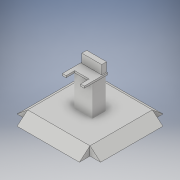
# Autodesk Inventor part: terminal stand removed rails 2nd map
Saved by Autodesk Inventor 2017 (Build 210142000, 142)
## iProperties
Created: 2018-03-07
Part Number: terminal stand removed rails 2nd map
Material: Generic
Document SubType Name: Modeling
Designer: Braxton
Density: 1 g/cm^3
Appearance: Default
Author: Braxton
Autodesk Inventor part; units mm, degrees
ref_plane "YZ Plane" through (0, 0, 0) normal (1, 0, 0) x (0, 1, 0)
ref_plane "bottom workplane" through (0, 0, 0) normal (0, 1, 0) x (-1, 0, 0)
ref_plane "XY Plane" through (0, 0, 0) normal (0, 0, 1) x (1, 0, 0)
sketch "bace of terminal" plane through (0, 0, 0) normal (0, 1, 0) x (-1, 0, 0)
  ellipse E0 centre (0, 0) end of major axis (25.4, 0) minor radius 19.05 construction
  line L0 (25.4, -19.05) -> (-25.4, -19.05)
  line L1 (-25.4, -19.05) -> (-25.4, 19.05)
  line L2 (-25.4, 19.05) -> (25.4, 19.05)
  line L3 (25.4, 19.05) -> (25.4, -19.05)
  point P0 (0, -19.05)
  dimension "d0" = 25.4
  dimension "d1" = 19.05
  constraints: 8 end point, 3 horizontal, 2 parallel, 2 vertical, 1 coincident, 1 perpendicular, 1 vertical alignment, 2 other
extrude "Extrusion16" add sketch "bace of terminal" along normal blind 92.6924
sketch "Sketch23" plane through (0, 92.6924, 0) normal (0, 1, 0) x (1, 0, 0)
  line L0 (0, 24.0896) -> (0, -74.4773) construction
  line L1 (-20.6375, -23.0226) -> (-31.2208, -23.0226) construction
  ellipse E0 centre (6.1023, 2.4529) end of major axis (37.558, 2.4529) minor radius 23.5917 (-25.2105, 0.2068) -> (-25.2085, 0.1915) ccw
  line L2 (20.6375, -23.0226) -> (31.2208, -23.0226) construction
  ellipse E1 centre (6.1023, 2.4529) end of major axis (-295.2488, 5.3941) minor radius 21.5528 (-0.0869, -19.0363) -> (0, -19.0372) ccw
  ellipse E2 centre (0, 0) end of major axis (25.3978, 0.4439) minor radius 19.0477
  line L3 (-25.9292, -47.625) -> (-25.9292, -19.05) construction
  line L4 (-25.9292, -19.05) -> (25.9292, -19.05) construction
  line L5 (3.3247, -11.6902) -> (-3.3534, -11.6902)
  line L6 (31.2208, 19.05) -> (-31.2208, 19.05)
  line L7 (-31.2208, 19.05) -> (-31.2208, -23.0226)
  line L8 (-25.4, 19.05) -> (-25.4, -19.05) projected
  line L9 (25.4, 19.05) -> (-25.4, 19.05) projected
  line L10 (25.4, -19.05) -> (25.4, 19.05) projected
  line L11 (-25.4, -19.05) -> (25.4, -19.05) projected
  line L12 (31.2208, -23.0226) -> (31.2208, 19.05)
  line L13 (-31.2208, -23.0226) -> (-31.2208, -47.625)
  line L14 (-31.2208, -47.625) -> (-20.6375, -47.625)
  line L15 (-20.6375, -47.625) -> (-20.6375, -23.0226)
  line L16 (31.2208, -23.0226) -> (31.2208, -47.625)
  line L17 (31.2208, -47.625) -> (20.6375, -47.625)
  line L18 (20.6375, -47.625) -> (20.6375, -23.0226)
  line L19 (-20.6375, -23.0226) -> (20.6375, -23.0226)
  point P0 (22.5643, 8.9693)
  dimension "d163" = 20.6375
  dimension "d165" = 10.5833
  dimension "d166" = 20.6375
  dimension "d167" = 10.5833
  dimension "d175" = 28.575
  dimension "d234" = 3.9726
  constraints: 32 end point, 9 vertical, 6 perpendicular, 5 horizontal, 4 collinear, 1 coincident, 1 midpoint, 1 point on line, 10 other
  measures "d163" distance from line of L1.start L0
  measures "d165" distance of L1.start L1.end
  measures "d166" distance from line of L2.start L0
  measures "d167" distance of L2.start L2.end
  measures "d175" distance of L3.start L3.end
  measures "d234" distance between parallel lines of L11 L1
extrude "arm rests and terminal monitor" add sketch "Sketch23" along normal blind 5.2917 separate body
ref_plane "middle of the part vertical" through (0, 0, 19.05) normal (1, 0, 0) x (0, 0, -1)
sketch "used to line up the key board and mouse" plane through (0, 97.984, 0) normal (0, 1, 0) x (1, 0, 0)
  line L0 (-25.9292, -46.3435) -> (-25.9292, -17.7685)
  line L1 (-25.9292, -17.7685) -> (25.9292, -17.7685) construction
  line L2 (25.9292, -46.1769) -> (25.9292, -17.7685)
  line L3 (-20.6375, -23.0226) -> (20.6375, -23.0226) projected
  point P0 (0, 0)
  dimension "d170" = 28.575
  dimension "d235" = 5.2541
  constraints: 6 end point, 1 horizontal, 1 perpendicular
  measures "d170" distance of L0.start L0.end
  measures "d235" distance between parallel lines of L3 L1
sketch "Sketch15" plane through (0, 0, 0) normal (0, -1, 0) x (1, 0, 0)
  line L0 (88.9, 88.9) -> (-88.9, 88.9)
  line L1 (-88.9, 88.9) -> (-88.9, -88.9)
  line L2 (-88.9, -88.9) -> (88.9, -88.9)
  line L3 (88.9, -88.9) -> (88.9, 88.9)
  line L4 (88.9, 0) -> (-88.9, 0) construction
  point P0 (0, 0)
  point P1 (0, 0)
  dimension "d236" = 177.8
  dimension "d237" = 177.8
  constraints: 10 end point, 3 midpoint, 2 parallel, 1 coincident, 1 horizontal, 1 perpendicular
  measures "d236" distance of L2.end L1.end
  measures "d237" distance of L1.end L0.end
extrude "bace" add sketch "Sketch15" along normal blind 25.4 bodies 2
sketch "Sketch31" plane through (88.9, 0, 88.9) normal (1, 0, 0) x (0, 0, -1)
  line L0 (0, 0) -> (0, -25.4) projected
  line L1 (0, 0) -> (0, -25.4)
  line L2 (0, -25.4) -> (-30.2705, -25.4)
  line L3 (-30.2705, -25.4) -> (0, 0)
  point P0 (88.9, 0)
  dimension "d238" = 40
  constraints: 6 end point, 1 perpendicular, 1 vertical
  measures "d238" angle of L2 L3
extrude "ramp to terminal" add sketch "Sketch31" against normal up to surface (177.8 mm away) bodies 2
pattern_circular "made rest of ramps to terminal" count 4 over 360 about axis through (0, -10, 0) along (0, 1, 0) of "ramp to terminal" bodies 2
ref_plane "mate to back to monitor" through (25.4, 0, -19.05) normal (0, 0, -1) x (-1, 0, 0)
sketch "Sketch25" plane through (0, 97.984, 0) normal (0, 1, 0) x (1, 0, 0)
  line L0 (0, 0) -> (0, 12.0948) construction
  line L1 (-31.2208, 19.05) -> (31.2208, 19.05) projected
  line L2 (28.3394, 5.0104) -> (-28.3394, 5.0104)
  line L3 (-28.3394, 5.0104) -> (-28.3394, 19.05)
  line L4 (-28.3394, 19.05) -> (28.3394, 19.05)
  line L5 (28.3394, 19.05) -> (28.3394, 5.0104)
  point P0 (0, 5.0104)
  dimension "d245" = 14.0396
  dimension "d246" = 56.6788
  dimension "d247" = 2.8814
  constraints: 10 end point, 2 parallel, 2 point on line, 1 horizontal, 1 perpendicular, 1 vertical
  measures "d245" distance of L4.end L2.start
  measures "d246" distance of L2.start L2.end
  measures "d247" distance from line of L1.end L5
extrude "monitor raise" add sketch "Sketch25" along normal blind 25.4 bodies 2
sketch "Sketch26" plane through (0, 0, 0) normal (0, 1, 0) x (1, 0, 0)
  line L0 (-2.9432, 29.9138) -> (2.9432, 29.9138)
  line L1 (2.9432, 29.9138) -> (2.9432, 20.32)
  line L2 (2.9432, 20.32) -> (-2.9432, 20.32)
  line L3 (-2.9432, 20.32) -> (-2.9432, 29.9138)
  line L4 (0, 19.05) -> (0, 20.32) construction
  line L5 (0, 0) -> (0, 19.05) construction
  line L6 (-25.4, 19.05) -> (25.4, 19.05) projected
  line L7 (25.4, -19.05) -> (-25.4, -19.05) projected
  line L8 (-25.4, 19.05) -> (25.4, 19.05)
  line L9 (25.4, 19.05) -> (25.4, -19.05)
  line L10 (25.4, -19.05) -> (-25.4, -19.05)
  line L11 (-25.4, -19.05) -> (-25.4, 19.05)
  line L12 (-25.4, 0) -> (0, 0)
  line L13 (0, 0) -> (0, -19.05)
  dimension "d182" = 5.8864
  dimension "d183" = 9.5938
  dimension "d185" = 1.27
  constraints: 24 end point, 4 midpoint, 4 parallel, 3 horizontal, 3 perpendicular, 2 vertical
  measures "d182" distance of L1.end L2.end
  measures "d183" distance of L0.end L1.end
  measures "d185" distance from line of L2 L4.start
ref_plane "Work Plane20" through (0, 0.4604, 0) normal (0, 1, 0) x (1, 0, 0)
sketch "Sketch27" plane through (0, 0.4604, 0) normal (0, 1, 0) x (1, 0, 0)
  line L0 (-2.4913, 29.4619) -> (2.4913, 29.4619)
  line L1 (2.4913, 29.4619) -> (2.4913, 20.7719)
  line L2 (2.4913, 20.7719) -> (-2.4913, 20.7719)
  line L3 (-2.4913, 20.7719) -> (-2.4913, 29.4619)
  line L4 (0, 0) -> (0, 19.05)
  line L5 (0, 19.05) -> (0, 20.7719) construction
  line L6 (-25.4, 19.05) -> (25.4, 19.05) projected
  point P0 (-25.4, 0)
  point P1 (-6.6832, 19.05)
  dimension "d186" = 1.7219
  dimension "d188" = 4.9826
  dimension "d189" = 8.69
  constraints: 12 end point, 2 midpoint, 2 parallel, 2 perpendicular, 1 coincident, 1 collinear, 1 horizontal, 1 point on line, 1 other
  measures "d186" distance from line of L2 L4.end
  measures "d188" distance between parallel lines of L1 L3
  measures "d189" distance between parallel lines of L2 L0
loft "outlet cap" add profiles "Sketch26", "Sketch27" bodies 2 contours L0 L1 L2 L3 / all
sketch "Sketch28" plane through (-2.4913, 0.4604, -29.4619) normal (0, 1, 0) x (1, 0, 0)
  line L0 (2.4913, -0.7892) -> (3.265, -0.7892)
  line L1 (2.4913, -3.1536) -> (3.265, -3.1536)
  arc A0 (3.265, -3.1536) -> (3.265, -0.7892) centre (2.4868, -1.9714) ccw
  line L2 (2.4913, -0.7892) -> (2.4913, -3.1536) construction
  line L3 (0, 0) -> (4.9826, 0) projected
  line L4 (2.4913, 0) -> (2.4913, 1.3195) construction
  line L5 (2.4913, -0.7892) -> (1.7177, -0.7892)
  line L6 (2.4913, -3.1536) -> (1.7177, -3.1536)
  arc A1 (1.7177, -0.7892) -> (1.7177, -3.1536) centre (2.4959, -1.9714) ccw
  line L7 (0, -8.69) -> (0, 0) projected
  line L8 (0, -4.345) -> (4.9826, -4.345) construction
  line L9 (2.4913, -7.9007) -> (3.265, -7.9007)
  line L10 (2.4913, -5.5364) -> (3.265, -5.5364)
  arc A2 (3.265, -7.9007) -> (3.265, -5.5364) centre (2.4868, -6.7186) ccw
  line L11 (2.4913, -7.9007) -> (2.4913, -5.5364) construction
  arc A3 (1.7177, -5.5364) -> (1.7177, -7.9007) centre (2.4959, -6.7186) ccw
  line L12 (2.4913, -5.5364) -> (1.7177, -5.5364)
  line L13 (2.4913, -7.9007) -> (1.7177, -7.9007)
  line L14 (1.9177, -1.3163) -> (2.032, -1.3163)
  line L15 (2.032, -1.3163) -> (2.032, -1.8455)
  line L16 (2.032, -1.8455) -> (1.9177, -1.8455)
  line L17 (1.9177, -1.8455) -> (1.9177, -1.3163)
  line L18 (3.0649, -1.3163) -> (2.9506, -1.3163)
  line L19 (2.9506, -1.3163) -> (2.9506, -1.8455)
  line L20 (2.9506, -1.8455) -> (3.0649, -1.8455)
  line L21 (3.0649, -1.8455) -> (3.0649, -1.3163)
  line L22 (2.4913, -2.7831) -> (2.6903, -2.7831)
  line L23 (2.6903, -2.7831) -> (2.6903, -2.5842)
  arc A4 (2.6903, -2.5842) -> (2.4913, -2.3852) centre (2.4913, -2.5842) ccw
  line L24 (2.4913, -2.7831) -> (2.2924, -2.7831)
  line L25 (2.2924, -2.7831) -> (2.2923, -2.5842)
  arc A5 (2.4913, -2.3852) -> (2.2923, -2.5842) centre (2.4913, -2.5842) ccw
  line L26 (1.9177, -6.0635) -> (2.032, -6.0635)
  line L27 (2.032, -6.0635) -> (2.032, -6.5926)
  line L28 (2.032, -6.5926) -> (1.9177, -6.5926)
  line L29 (1.9177, -6.5926) -> (1.9177, -6.0635)
  line L30 (3.0649, -6.0635) -> (2.9506, -6.0635)
  line L31 (2.9506, -6.0635) -> (2.9506, -6.5926)
  line L32 (3.0649, -6.5926) -> (3.0649, -6.0635)
  line L33 (2.9506, -6.5926) -> (3.0649, -6.5926)
  line L34 (2.4913, -7.5303) -> (2.6903, -7.5303)
  line L35 (2.6903, -7.5303) -> (2.6903, -7.3313)
  arc A6 (2.6903, -7.3313) -> (2.5559, -7.1432) centre (2.4913, -7.3313) ccw
  arc A7 (2.5559, -7.1432) -> (2.2924, -7.3313) centre (2.4913, -7.3313) ccw
  line L36 (2.2924, -7.5303) -> (2.2924, -7.3313)
  line L37 (2.4913, -7.5303) -> (2.2924, -7.5303)
  point P0 (2.4913, -29.4619)
  point P1 (3.9021, -1.9714)
  point P2 (1.0806, -1.9714)
  point P3 (3.9021, -6.7186)
  point P4 (1.0806, -6.7186)
  dimension "d194" = 0.6371
  dimension "d195" = 0.7736
  dimension "d197" = 2.3643
  dimension "d198" = 0.7893
  dimension "d199" = 0.9186
  dimension "d200" = 0.1143
  dimension "d201" = 0.5292
  dimension "d202" = 0.5271
  dimension "d203" = 0.199
  dimension "d204" = 0.7387
  dimension "d205" = 0.199
  dimension "d206" = 0.9186
  dimension "d207" = 0.1143
  dimension "d208" = 0.5292
  dimension "d209" = 0.199
  dimension "d211" = 0.199
  dimension "d212" = 0.5271
  dimension "d213" = 0.4593
  dimension "d214" = 0.7387
  constraints: 72 end point, 21 symmetric about line, 17 point on circle, 8 centre point, 8 horizontal, 5 perpendicular, 5 tangent, 4 equal length, 4 parallel, 3 collinear, 3 point on line, 2 midpoint, 1 concentric, 1 vertical, 4 other
  measures "d194" horizontal distance of L0.end point (3.902, -1.971)
  measures "d195" distance of L0.start L0.end
  measures "d197" distance between parallel lines of L1 L0
  measures "d198" distance between parallel lines of L0 L3
  measures "d199" distance between parallel lines of L19 L15
  measures "d200" distance of L14.start L14.end
  measures "d201" distance between parallel lines of L14 L16
  measures "d202" distance between parallel lines of L5 L14
  measures "d203" radius of A5
  measures "d204" distance from line of L16 A4.centre
  measures "d205" distance from line of L22 A4.centre
  measures "d206" distance between parallel lines of L31 L27
  measures "d207" distance of L29.end L27.start
  measures "d208" distance between parallel lines of L26 L28
  measures "d209" radius of A7
  measures "d211" distance from line of L34 A6.centre
  measures "d212" distance between parallel lines of L12 L26
  measures "d213" distance between parallel lines of L31 L11
  measures "d214" distance from line of L28 A6.centre
extrude "outlet revele out" add sketch "Sketch28" along normal blind 0.0762 bodies 2
extrude "hot and ground wire holes" cut sketch "Sketch28" against normal blind 1.6478 contours L14 L15 L16 L17 | L21 L20 L19 L18 | L24 L25 A5 A4 L23 L22 | L26 L27 L28 L29 | L32 L33 L31 L30 | L37 L36 A7 A6 L35 L34 bodies 2
ref_plane "screw workplane" through (-2.4913, 0.4604, -25.1169) normal (0, 0, 1) x (1, 0, 0)
sketch "Sketch29" plane through (-2.4913, 0.4604, -25.1169) normal (0, 0, 1) x (1, 0, 0)
  line L0 (3.265, 0) -> (1.7177, 0) projected
  line L1 (2.4913, 0) -> (2.2167, 0)
  line L2 (2.4913, 0) -> (2.4913, 0.0698)
  arc A0 (2.4913, 0.0698) -> (2.2167, 0) centre (2.4913, -0.505) ccw
  line L3 (2.4913, 0.0698) -> (2.567, 0.0698) construction
  point P0 (2.4913, -0.4604)
  dimension "d226" = 0.2746
  dimension "d227" = 0.0698
  constraints: 6 end point, 2 point on circle, 1 centre point, 1 horizontal, 1 midpoint, 1 perpendicular, 1 point on line, 1 tangent
  measures "d226" distance of L1.start L1.end
  measures "d227" distance of L1.start L2.end
revolve "screw made" add sketch "Sketch29" angle 360 about axis through (0, 0.4604, -25.1169) along (0, 1, 0) bodies 2
sketch "Sketch30" plane through (-2.4913, 0.4604, -29.4619) normal (0, 1, 0) x (1, 0, 0)
  line L0 (0, -8.69) -> (0, 0) projected
  line L1 (4.9826, 0) -> (4.9826, -8.69) projected
  circle A0 centre (2.4913, -4.345) radius 0.2746 projected
  line L2 (2.4913, -4.345) -> (2.4913, -4.0703) construction
  line L3 (2.2167, -4.345) -> (2.766, -4.345) construction
  line L4 (2.4527, -4.345) -> (2.4527, -4.0731)
  arc A1 (2.4913, -4.0703) -> (2.4527, -4.0731) centre (2.4913, -4.345) ccw
  line L5 (2.5299, -4.345) -> (2.5299, -4.0731)
  arc A2 (2.5299, -4.0731) -> (2.4913, -4.0703) centre (2.4913, -4.345) ccw
  line L6 (2.4527, -4.345) -> (2.4527, -4.6169)
  arc A3 (2.4527, -4.6169) -> (2.4913, -4.6196) centre (2.4913, -4.345) ccw
  line L7 (2.5299, -4.345) -> (2.5299, -4.6169)
  arc A4 (2.4913, -4.6196) -> (2.5299, -4.6169) centre (2.4913, -4.345) ccw
  point P0 (2.4913, -29.4619)
  dimension "d229" = 0.0386
  constraints: 12 end point, 12 point on circle, 5 symmetric about line, 4 centre point, 1 concentric, 1 parallel, 1 perpendicular, 1 point on line, 1 vertical, 3 other
  measures "d229" distance between parallel lines of L2 L4
extrude "slot for screw" cut sketch "Sketch30" along normal mid plane 0.326 contours L5 L7 A0 L6 L4 bodies 2
equation "\"d43\" = d50"
equation "\"d50\" = 21.59"
body "Solid4"
